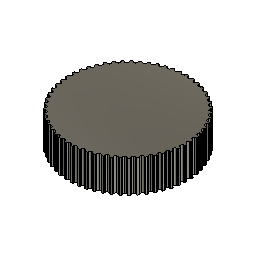
gear_59z (Autodesk Fusion 360 design; units mm, degrees)
Autodesk Fusion 360 part; units mm, degrees
sketch "Sketch1" plane through (0, 0, 0) normal (0, 0, 1) x (1, 0, 0) in component "gt2 pulley"
  circle A0 centre (0, 0) radius 18.7803 construction
  circle A1 centre (0, 0) radius 17.7763 construction
  line L0 (0, 0) -> (0, 18.7803) construction
  line L1 (0, 0) -> (0.9995, 18.7537) construction
  line L2 (0, 0) -> (1.4063, 18.7276) construction
  circle A2 centre (0, 0) radius 18.5263 construction
  arc A3 (0.3911, 18.3877) -> (0.4622, 18.0946) centre (1.3873, 18.4743) ccw
  circle A4 centre (0, 0) radius 18.3763 construction
  arc A5 (0.2435, 18.5247) -> (0, 18.5263) centre (0, 0) ccw
  arc A6 (0.3911, 18.3877) -> (0.2435, 18.5247) centre (0.2416, 18.3747) ccw
  arc A7 (0.4622, 18.0946) -> (0.9461, 17.7511) centre (0.9756, 18.3053) ccw
  arc A8 (0, 18.5263) -> (-0.2435, 18.5247) centre (0, 0) ccw
  arc A9 (-0.2435, 18.5247) -> (-0.3911, 18.3877) centre (-0.2416, 18.3747) ccw
  arc A10 (-0.4622, 18.0946) -> (-0.3911, 18.3877) centre (-1.3873, 18.4743) ccw
  arc A11 (-0.9461, 17.7511) -> (-0.4622, 18.0946) centre (-0.9756, 18.3053) ccw
  arc A12 (0.9461, 17.7511) -> (-0.9461, 17.7511) centre (0, 0) ccw
  point P0 (1.3873, 18.4743)
  point P1 (0, 18.5263)
  dimension "d18" = 37.5606
  dimension "d19" = 3.051
  dimension "d22" = 1.004
  dimension "d24" = 0.75
  dimension "d26" = 1
  dimension "d27" = 0.15
  dimension "d28" = 0.15
  dimension "d47" = 0.555
  dimension "d52" = 3.812
  constraint coincident A0.centre A1.centre
  constraint coincident A0 L0.end
  constraint vertical L0
  constraint coincident A0 L1.end
  constraint coincident A0 L2.end
  constraint concentric A1 A2
  constraint coincident A1 A7.end
  constraint coincident L1 A7.end
  constraint coincident A2 P0
  constraint coincident L2 P0
  constraint coincident P0 A3.centre
  constraint coincident A2 P1
  constraint coincident L0 P1
  constraint concentric A2 A4
  constraint coincident P1 A5.end
  constraint coincident A4 A6.centre
  constraint coincident A3.start A6.start
  constraint tangent A3 A6
  constraint tangent A3 A7
  constraint symmetric L0 A7.end A11.start
  constraint symmetric L0 A3.start A9.end
  constraint symmetric L0 A3.end A10.start
  constraint symmetric L0 A3 A10
  constraint symmetric L0 A5.start A8.end
  constraint symmetric L0 P1 A5.end
  constraint symmetric L0 A5 A8
  constraint symmetric L0 A6 A9
  constraint symmetric L0 A7 A11
  constraint coincident A1 A11.start
  constraint tangent A1 A7
  constraint coincident L1 A7.centre
  measures "d18" diameter of A0
  measures "d19" angle of L0 L1
  measures "d22" distance of A0 A1
  measures "d24" distance of A1 A2
  measures "d26" radius of A3
  measures "d27" distance of A2 A4
  measures "d28" radius of A6
  measures "d47" radius of A7
extrude "Extrude1" add sketch "Sketch1" along normal blind 10 makes body 1
pattern_circular "C-Pattern1" count 59 over 360 about axis through (0, 0, 1.75) along (0, 0, 1) of bodies 1 makes body 2 at (-1.1561, 17.7387, 3.3333) makes body 3 at (-4.4737, 17.2041, 6.6667) makes body 4 at (-5.6829, 16.8434, 6.6667) makes body 5 at (-6.6689, 16.4779, 3.3333) makes body 6 at (-9.6508, 14.9285, 6.6667) makes body 7 at (-10.0013, 14.6959, 3.3333) makes body 8 at (-12.5883, 12.5511, 6.6667) makes body 9 at (-13.4469, 11.6265, 6.6667) makes body 10 at (-14.9569, 9.6066, 6.6667) makes body 11 at (-15.8933, 7.9623, 6.6667) makes body 12 at (-16.4181, 6.8148, 6.6667) makes body 13 at (-17.0495, 5.0311, 6.6667) makes body 14 at (-17.3171, 4.0142, 3.3333) makes body 15 at (-17.7277, 1.3134, 6.6667) makes body 16 at (-17.7669, -0.5783, 6.6667) makes body 17 at (-17.7016, -1.6279, 3.3333) makes body 18 at (-17.4283, -3.5002, 3.3333) makes body 19 at (-16.4581, -6.7176, 6.6667) makes body 20 at (-15.6509, -8.4289, 6.6667) makes body 21 at (-15.447, -8.7969, 3.3333) makes body 22 at (-13.5155, -11.5468, 6.6667) makes body 23 at (-12.6623, -12.4764, 6.6667) makes body 24 at (-11.2644, -13.7517, 6.6667) makes body 25 at (-9.7389, -14.8711, 6.6667) makes body 26 at (-8.8426, -15.4209, 3.3333) makes body 27 at (-5.7824, -16.8095, 6.6667) makes body 28 at (-4.5754, -17.1774, 6.6667) makes body 29 at (-2.7237, -17.5664, 6.6667) makes body 30 at (-1.6802, -17.6967, 3.3333) makes body 31 at (1.0511, -17.7452, 6.6667) makes body 32 at (2.3072, -17.6259, 6.6667) makes body 33 at (5.383, -16.9416, 6.6667) makes body 34 at (6.5713, -16.5171, 6.6667) makes body 35 at (8.8426, -15.4209, 6.6667) makes body 36 at (9.205, -15.2074, 3.3333) makes body 37 at (10.7693, -14.1428, 3.3333) makes body 38 at (12.8091, -12.3257, 6.6667) makes body 39 at (14.3005, -10.5589, 6.6667) makes body 40 at (15.447, -8.7969, 6.6667) makes body 41 at (15.6509, -8.4289, 3.3333) makes body 42 at (16.4581, -6.7176, 3.3333) makes body 43 at (17.0789, -4.9301, 3.3333) makes body 44 at (17.6327, -2.2551, 6.6667) makes body 45 at (17.7725, -0.3681, 6.6667) makes body 46 at (17.7109, 1.5231, 6.6667) makes body 47 at (17.4487, 3.397, 6.6667) makes body 48 at (17.2173, 4.4228, 3.3333) makes body 49 at (16.0773, 7.584, 6.6667) makes body 50 at (15.1801, 9.2499, 6.6667) makes body 51 at (14.9569, 9.6066, 3.3333) makes body 52 at (12.8818, 12.2497, 6.6667) makes body 53 at (11.9804, 13.1327, 6.6667) makes body 54 at (10.0013, 14.6959, 6.6667) makes body 55 at (9.6508, 14.9285, 3.3333) makes body 56 at (7.2495, 16.2309, 6.6667) makes body 57 at (5.4832, 16.9095, 6.6667) makes body 58 at (3.6547, 17.3965, 6.6667) makes body 59 at (1.7849, 17.6864, 6.6667)
sketch "Sketch2" plane through (0, 0, 10) normal (0, 0, 1) x (-1, 0, 0)
  arc A0 (-11.2797, -14.5268) -> (-11.243, -14.7247) centre (-11.152, -14.6055) ccw
  arc A1 (-11.243, -14.7247) -> (-10.852, -15.0152) centre (0, 0) ccw
  arc A2 (-10.852, -15.0152) -> (-10.6519, -14.9932) centre (-10.7641, -14.8937) ccw
  arc A3 (-10.42, -14.8004) -> (-10.6519, -14.9932) centre (-9.9038, -15.6569) ccw
  arc A4 (-9.8267, -14.8132) -> (-10.42, -14.8004) centre (-10.1335, -15.2757) ccw
  arc A5 (-11.3456, -13.6848) -> (-9.8267, -14.8132) centre (0, 0) ccw
  arc A6 (-11.162, -14.2491) -> (-11.3456, -13.6848) centre (-11.6998, -14.112) ccw
  arc A7 (-11.2797, -14.5268) -> (-11.162, -14.2491) centre (-12.1311, -14.0022) ccw
  circle A8 centre (0, 0) radius 17.7763
  constraint concentric A1 A8
extrude "Extrude2" add sketch "Sketch2" against normal blind 10 contours A5 A8 bodies 1 2 3 4 5 6 7 8 9 10 11 12 13 14 15 16 17 18 19 20 21 22 23 24 25 26 27 28 29 30 31 32 33 34 35 36 37 38 39 40 41 42 43 44 45 46 47 48 49 50 51 52 53 54 55 56 57 58 59
extrude "Extrude4" [suppressed] in component "gt2 pulley"
pattern_circular "C-Pattern7" [suppressed] in component "gt2 pulley"
extrude "Extrude3" [suppressed] in component "gt2 pulley"
pattern_circular "C-Pattern6" [suppressed] in component "gt2 pulley"
extrude "Extrude2'" [suppressed] in component "gt2 pulley"
pattern_circular "C-Pattern5" [suppressed] in component "gt2 pulley"
extrude "Extrude1'" [suppressed] in component "gt2 pulley"
pattern_circular "C-Pattern4" [suppressed] in component "gt2 pulley"
pattern_circular "C-Pattern3" [suppressed] in component "gt2 pulley"
pattern_circular "C-Pattern2" [suppressed] in component "gt2 pulley"
pattern_circular "C-Pattern1'" [suppressed] in component "gt2 pulley"
copy_body "Body->Comp1" [suppressed] in component "Component"
copy_body "Body->Comp2" [suppressed] in component "Component'"
copy_body "Body->Comp3" [suppressed] in component "Component''"
copy_body "Body->Comp4" [suppressed] in component "Component'''"
copy_body "Body->Comp5" [suppressed] in component "Component''''"
copy_body "Body->Comp6" [suppressed] in component "Component'''''"
copy_body "Body->Comp7" [suppressed] in component "Component''''''"
copy_body "Body->Comp8" [suppressed] in component "Component'''''''"
copy_body "Body->Comp9" [suppressed] in component "Component''''''''"
copy_body "Body->Comp10" [suppressed] in component "Component'''''''''"
copy_body "Body->Comp11" [suppressed] in component "Component''''''''''"
copy_body "Body->Comp12" [suppressed] in component "Component'''''''''''"
copy_body "Body->Comp13" [suppressed] in component "Component''''''''''''"
copy_body "Body->Comp14" [suppressed] in component "Component'''''''''''''"
copy_body "Body->Comp15" [suppressed] in component "Component''''''''''''''"
copy_body "Body->Comp16" [suppressed] in component "Component'''''''''''''''"
copy_body "Body->Comp17" [suppressed] in component "Component''''''''''''''''"
copy_body "Body->Comp18" [suppressed] in component "Component'''''''''''''''''"
copy_body "Body->Comp19" [suppressed] in component "Component''''''''''''''''''"
copy_body "Body->Comp20" [suppressed] in component "Component'''''''''''''''''''"
component "gt2 pulley" placed x (1, 0, 0) y (0, 1, 0) z (0, 0, 1) at (0, 0, 0)
equation "NumTeeth = 59" comment "min 20"
equation "ToothPitch = 2 mm"
equation "PullyDia = NumTeeth * ToothPitch / PI"
equation "ToothAng = ( ( 360 / NumTeeth ) * 1 deg )"
equation "TransOffsetAngle = ToothAng * 0.2"
equation "Sholulder_Radius = 0.15 mm"
equation "Root_Radius = 0.555 mm"
equation "TransRadius = 1 mm"
equation "ToolHeight = 0.75 mm"
equation "PLD = 0.254 mm"
equation "d18 = PullyDia"
equation "d19 = ToothAng / 2"
equation "d22 = PLD + ToolHeight"
equation "d24 = ToolHeight"
equation "d26 = TransRadius"
equation "d27 = Sholulder_Radius"
equation "d31 = NumTeeth"
equation "d33 = NumTeeth"
equation "d35 = NumTeeth"
equation "d37 = NumTeeth"
equation "d41 = NumTeeth"
equation "d45 = NumTeeth"
equation "d47 = Root_Radius"
equation "d50 = NumTeeth"
